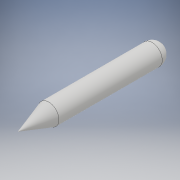
# Autodesk Inventor part: parametrized pencile
Saved by Autodesk Inventor 2017 (Build 210142000, 142)
## iProperties
Created: 2016-12-05
Part Number: parametrized pencile
Material: Generic
Document SubType Name: Modeling
Designer: ycsev
Density: 1 g/cm^3
Appearance: Default
Author: ycsev
Autodesk Inventor part; units mm, degrees
ref_plane "YZ Plane" through (0, 0, 0) normal (1, 0, 0) x (0, 1, 0)
ref_plane "XZ Plane" through (0, 0, 0) normal (0, 1, 0) x (-1, 0, 0)
ref_plane "XY Plane" through (0, 0, 0) normal (0, 0, 1) x (1, 0, 0)
sketch "Sketch1" plane through (0, 0, 0) normal (0, 1, 0) x (-1, 0, 0)
  circle A0 centre (0, 0) radius 5
  dimension "d0" = 10
  constraints: 1 centre point, 1 coincident
  measures "d0" diameter of A0
extrude "Extrusion1" add sketch "Sketch1" along normal blind 50
sketch "Sketch2" plane through (0, 0, 0) normal (1, 0, 0) x (0, 1, 0)
  line L0 (0, 5) -> (0, -5) projected
  line L1 (0, -5) -> (0, 0)
  line L2 (-15, 0) -> (0, 0)
  line L3 (0, -5) -> (-15, 0)
  dimension "d3" = 15
  constraints: 6 end point, 1 midpoint, 1 perpendicular, 1 point on line
  measures "d3" distance of L2.start L1.end
revolve "Revolution1" add sketch "Sketch2" angle 360 about axis through (0, -15, 0) along (0, 1, 0)
sketch "Sketch4" plane through (0, 0, 0) normal (1, 0, 0) x (0, 1, 0)
  line L0 (50, -5) -> (50, 5) projected
  arc A0 (50, -5) -> (55, 0) centre (50, 0) ccw
  line L1 (55, 0) -> (50, 0)
  line L2 (50, -5) -> (50, 0)
  point P0 (0, 0)
  constraints: 4 end point, 2 point on circle, 1 centre point, 1 horizontal, 1 midpoint, 1 perpendicular
revolve "Revolution2" add sketch "Sketch4" angle 360 about axis through (0, 55, 0) along (0, -1, 0)
equation "\"d0\" = cylinder_r"
equation "\"d1\" = cylinder_h"
equation "\"d3\" = cone_h"
equation "\"cylinder_h\" = 50"
equation "\"cone_h\" = 15"
equation "\"cylinder_r\" = 10"
body "Solid1"
